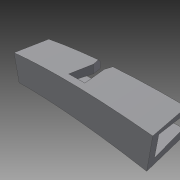
# Autodesk Inventor part: HanesBand-Adjuster
Saved by Autodesk Inventor 2015 (Build 190159000, 159)
## iProperties
Created: 2020-03-26
Part Number: HanesBand-Adjuster
Material: Generic
Document SubType Name: Modeling
Designer: Dominick Lee
Density: 1 g/cm^3
Appearance: Default
Author: Dominick Lee
Autodesk Inventor part; units mm, degrees
ref_plane "YZ Plane" through (0, 0, 0) normal (1, 0, 0) x (0, 1, 0)
ref_plane "XZ Plane" through (0, 0, 0) normal (0, 1, 0) x (-1, 0, 0)
ref_plane "XY Plane" through (0, 0, 0) normal (0, 0, 1) x (1, 0, 0)
sketch "Sketch1" plane through (0, 0, 0) normal (0, 1, 0) x (-1, 0, 0)
  line L0 (12.5, 3) -> (-12.5, 3)
  line L1 (-12.5, 3) -> (-12.5, -3)
  line L2 (-12.5, -3) -> (12.5, -3)
  line L3 (12.5, -3) -> (12.5, 3)
  line L4 (12.5, 3) -> (-12.5, -3) construction
  line L5 (-12.5, 3) -> (12.5, -3) construction
  point P0 (0, 0)
  dimension "d0" = 25
  dimension "d1" = 6
  constraints: 12 end point, 2 midpoint, 2 parallel, 1 horizontal, 1 perpendicular
  measures "d0" distance of L0.start L0.end
  measures "d1" distance of L1.end L0.end
extrude "Extrusion1" add sketch "Sketch1" along normal blind 1.2
sketch "Sketch2" plane through (0, 1.2, 0) normal (0, 1, 0) x (1, 0, 0)
  line L0 (-12.5, 3) -> (12.5, 3)
  line L1 (12.5, 3) -> (12.5, 1.8)
  line L2 (12.5, 1.8) -> (-12.5, 1.8)
  line L3 (-12.5, 1.8) -> (-12.5, 3)
  line L4 (12.5, -3) -> (12.5, -1.8)
  line L5 (-12.5, -1.8) -> (-12.5, -3)
  line L6 (-1.5, -3) -> (-1.5, -1.8)
  line L7 (1.5, -1.8) -> (1.5, -3)
  line L8 (-1.5, -3) -> (1.5, -1.8) construction
  line L9 (-1.5, -1.8) -> (1.5, -3) construction
  line L10 (12.5, -1.8) -> (1.5, -1.8)
  line L11 (-1.5, -1.8) -> (-12.5, -1.8)
  line L12 (-12.5, -3) -> (-1.5, -3)
  line L13 (1.5, -3) -> (12.5, -3)
  point P0 (0, 0)
  point P1 (0, -2.4)
  dimension "d13" = 1.2
  dimension "d14" = 1.2
  dimension "d15" = 3
  constraints: 28 end point, 8 parallel, 3 horizontal, 3 perpendicular, 2 midpoint, 1 other
  measures "d13" distance of L0.end L1.end
  measures "d14" distance of L4.end L4.start
  measures "d15" distance of L6.end L7.start
extrude "Extrusion3" add sketch "Sketch2" along normal blind 6
sketch "Sketch4" plane through (-12.5, 0, 3) normal (0, 0, 1) x (1, 0, 0)
  line L0 (11, 7.2) -> (11.5176, 5.2681)
  line L1 (11, 7.2) -> (13, 7.2) construction
  line L2 (11.5176, 5.2681) -> (11, 1.2)
  line L3 (11, 1.2) -> (11, 7.2)
  line L4 (14, 7.2) -> (13.4824, 5.2681)
  line L5 (14, 7.2) -> (16, 7.2) construction
  line L6 (13.4824, 5.2681) -> (14, 1.2)
  line L7 (14, 1.2) -> (14, 7.2)
  point P0 (12.5, 0)
  dimension "d18" = 2
  dimension "d19" = 75
  dimension "d20" = 2
  dimension "d21" = 105
  constraints: 16 end point, 2 equal length, 2 horizontal, 2 vertical
  measures "d18" distance of L0.start L0.end
  measures "d19" angle of L0 L1
  measures "d20" distance of L4.start L4.end
  measures "d21" angle of L4 L5
extrude "Extrusion4" add sketch "Sketch4" against normal blind 1.2
draft "FaceDraft1" angle 5 pull direction (0, -1, 0) faces at (4.1667, 3.2, -1.8) fixed edges at (0, 1.2, -1.8)
draft "FaceDraft2" angle 5 pull direction (0, -1, 0) faces at (8.6608, 4.556, 1.8) fixed edges at (7, 1.2, 1.8)
draft "FaceDraft3" angle 5 pull direction (0, -1, 0) faces at (-8.6608, 4.556, 1.8) fixed edges at (-7, 1.2, 1.8)
sketch "Sketch5" plane through (0, 7.2, 0) normal (0, 1, 0) x (1, 0, 0)
  line L0 (12.5, 3) -> (-12.5, 3) projected
  line L1 (0, 3) -> (0, 2.4)
  arc A0 (-12.5, 3) -> (12.5, 3) centre (0, 132.9083) ccw
  line L2 (1.5, -3) -> (-1.5, -3)
  line L3 (0, -3) -> (0, -2.4)
  line L4 (-12.5, -1.2751) -> (-12.5, -3) projected
  line L5 (12.5, -3) -> (12.5, -1.2751) projected
  arc A1 (-12.5, -2.4) -> (12.5, -2.4) centre (0, 127.5083) ccw
  line L6 (12.5, -2.4) -> (12.5, -3.3805)
  line L7 (12.5, -3.3805) -> (-12.5, -3.3805)
  line L8 (-12.5, -3.3805) -> (-12.5, -2.4)
  point P0 (0, 0)
  dimension "d27" = 0.6
  dimension "d30" = 0.6
  constraints: 12 end point, 6 point on circle, 4 vertical, 2 centre point, 2 horizontal, 2 midpoint, 2 point on line
  measures "d27" distance of L1.start L1.end
  measures "d30" distance of L3.start L3.end
extrude "Extrusion5" cut sketch "Sketch5" against normal blind 7.45
chamfer "Chamfer1" distance 0.6 angle 45 2 edges at (-7.0062, 7.2, 2.8118) (7.0062, 7.2, 2.8118)
body "Solid1"
